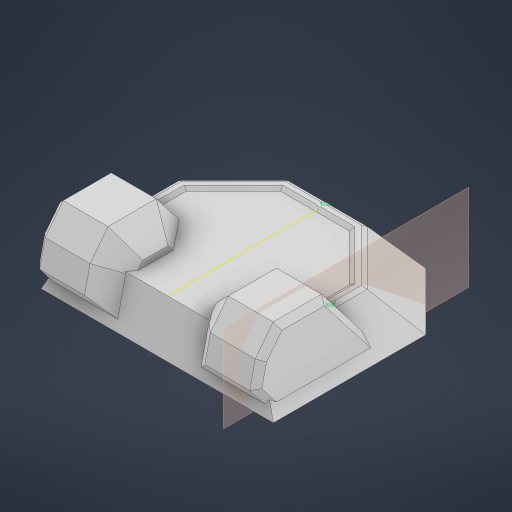
# Autodesk Inventor part: chassis
Saved by Autodesk Inventor 2023 (Build 270158000, 158)
## iProperties
Created: 2022-06-22
Part Number: chassis
Material: Generic
Document SubType Name: Modeling
Designer: Dan
Density: 1 g/cm^3
Appearance: Default
Author: Dan
Autodesk Inventor part; units mm, degrees
ref_plane "XY Plane" through (0, 0, 0) normal (0, 0, 1) x (1, 0, 0)
sketch "Sketch2" plane through (0, 0, 0) normal (0, 1, 0) x (-1, 0, 0)
  line L0 (0, -90) -> (0, 90)
  line L1 (0, -90) -> (-50, -90)
  line L2 (-50, -90) -> (-99.4975, -40.5025)
  line L3 (-99.4975, -40.5025) -> (-99.4975, 90)
  line L4 (-99.4975, 90) -> (0, 90)
  point P0 (0, 0)
  dimension "d0" = 180
  dimension "d1" = 50
  dimension "d2" = 70
  dimension "d3" = 135
  constraints: 10 end point, 2 midpoint, 2 perpendicular, 1 horizontal, 1 vertical
  measures "d0" distance of L0.start L0.end
  measures "d1" distance of L0.start L1.end
  measures "d2" distance of L1.end L2.end
  measures "d3" angle of L1 L2
ref_plane "Top" through (0, 40, 0) normal (0, 1, 0) x (-1, 0, 0)
sketch "Sketch3" plane through (0, 40, 0) normal (0, 1, 0) x (-1, 0, 0)
  line L0 (0, -90) -> (0, 90) projected
  line L1 (0, -90) -> (-50, -90) projected
  line L2 (-50, -90) -> (-99.4975, -40.5025) projected
  line L3 (-99.4975, -40.5025) -> (-99.4975, 90) projected
  line L4 (-99.4975, 90) -> (0, 90) projected
  line L5 (-34.0658, -55.9075) -> (0, -55.9075)
  line L6 (0, 81.0844) -> (-80.6502, 81.0844)
  line L7 (-80.6502, 81.0844) -> (-80.6502, -9.3231)
  line L8 (-80.6502, -9.3231) -> (-34.0658, -55.9075)
  point P0 (0, 0)
  constraints: 8 end point, 4 parallel, 2 point on line, 1 horizontal, 1 vertical
loft "Loft1" add profiles "Sketch2", "Sketch3" contours all / L5 L8 L7 L6 L0
ref_plane "WHeel" through (60, 0, -90) normal (-1, 0, 0) x (0, 0, 1)
sketch "Sketch4" plane through (60, 0, -90) normal (-1, 0, 0) x (0, 0, 1)
  line L0 (49.4975, 0) -> (180, 0) projected
  line L1 (150, -2) -> (150, 63) construction
  circle A0 centre (150, 30.5) radius 32.5
  point P0 (90, 0)
  dimension "wheeld" = 65
  dimension "rideh" = 2
  dimension "d14" = 65
  dimension "d17" = 30
  constraints: 2 end point, 1 centre point, 1 midpoint, 1 vertical
  measures "wheeld" distance of L1.start L1.end
  measures "rideh" distance from line of L1.start L0
  measures "d14" diameter of A0
  measures "d17" distance from line of L0.end L1
extrude "Extrusion1" add sketch "Sketch4" against normal blind 35 separate body
sketch "Sketch5" plane through (95, 30.5, 60) normal (1, 0, 0) x (0, 0, -1)
  circle A0 centre (0, 0) radius 32.5 projected
  line L0 (-20.6148, 34.967) -> (20.6148, 34.967)
  line L1 (20.6148, 34.967) -> (71.6455, -30.5)
  line L2 (-30, -30.5) -> (100.5025, -30.5) projected
  line L3 (100.5025, -30.5) -> (69.3231, 9.5) projected
  circle A1 centre (0, 0) radius 32.5 projected
  line L4 (0, 32.5) -> (0, 40.0339) construction
  line L5 (-20.6148, 34.967) -> (-36.015, 15.2102)
  line L6 (-40.7271, -5.9307) -> (-21.5757, -30.5)
  line L7 (-36.015, 15.2102) -> (-40.7271, -5.9307)
  line L8 (-41.2569, -30.5) -> (-31.8085, 11.8903) projected
  line L9 (71.6455, -30.5) -> (-21.5757, -30.5)
  point P0 (60, -30.5)
  point P1 (0, 34.967)
  point P2 (-21.0844, 9.5)
  dimension "d18" = 127.936
  dimension "d19" = 127.936
  constraints: 14 end point, 4 point on line, 2 parallel, 1 collinear, 1 horizontal, 1 midpoint, 1 vertical, 1 vertical alignment, 1 other
  measures "d18" angle of L0 L1
  measures "d19" angle of L5 L0
extrude "Extrusion2" add sketch "Sketch5" against normal blind 63.5 separate body contours A0 L2 | A0 L2 L6 L7 L5 L0 L1 picked at (-8.2922, 7.0851)
chamfer "Chamfer1" distance 20 angle 45 4 edges at (31.5, 32.7335, 13.8699) (31.5, 65.467, 60) (31.5, 35.1397, 98.371) (31.5, 55.5886, 88.3149)
chamfer "Chamfer2" distance 5 angle 45 5 edges at (95, 32.7335, 13.8699) (95, 65.467, 60) (95, 55.5886, 88.3149) (95, 35.1397, 98.371) (95, 12.2846, 91.1514)
ref_plane "Work Plane3" through (0, 42, 81.0844) normal (0, 1, 0) x (1, 0, 0)
sketch "Sketch7" plane through (0, 42, 81.0844) normal (0, 1, 0) x (1, 0, 0)
  line L0 (34.0658, 136.9919) -> (0, 136.9919) projected
  line L1 (80.6502, 90.4075) -> (34.0658, 136.9919) projected
  line L2 (80.6502, 0) -> (80.6502, 90.4075) projected
  line L3 (0, 0) -> (80.6502, 0) projected
  line L4 (31.9947, 131.9919) -> (77.6502, 86.3364)
  line L5 (77.6502, 86.3364) -> (77.6502, 3)
  line L6 (77.6502, 3) -> (0, 3)
  line L7 (31.9947, 131.9919) -> (0, 131.9919)
  line L8 (0, 171.0844) -> (0, -8.9156) projected
  line L9 (0, 136.9919) -> (0, 0) projected
  point P0 (0, 81.0844)
  dimension "d37" = 5
  dimension "d38" = 5
  dimension "d39" = 3
  constraints: 8 end point, 1 parallel, 1 other
  measures "d37" distance between parallel lines of L1 L4
  measures "d38" distance between parallel lines of L0 L7
  measures "d39" distance between parallel lines of L2 L5
sketch "Sketch6" plane through (31.5, 30.5, 60) normal (-1, 0, 0) x (0, 0, 1)
  line L0 (-46.2872, -30.5) -> (21.5757, -30.5) projected
  line L1 (17.4734, 6.4652) -> (24.7927, -26.3729) projected
  line L2 (-10.8463, 14.967) -> (10.8463, 14.967) projected
  line L3 (-46.2872, -30.5) -> (-10.8463, 14.967) projected
  line L4 (-46.2872, -30.5) -> (21.5757, -30.5) projected
  line L5 (21.5757, -30.5) -> (24.7927, -26.3729) projected
  line L6 (10.8463, 14.967) -> (17.4734, 6.4652) projected
  point P0 (-60, -30.5)
  point P1 (-46.2872, -30.5)
extrude "Extrusion3" [suppressed]
combine bodies "Combine1" operation type add bodies to combine 3 1
shell "Shell1" thickness 3 removed faces 1 at (0, 3.3333, 15.7504) bodies 3
sketch "Sketch8" plane through (0, 0, -90) normal (-1, 0, 0) x (0, 0, 1)
  line L0 (80.6769, 40) -> (34.0925, 40) projected
  line L1 (34.0925, 40) -> (37.5566, 42)
  line L2 (41.5566, 42) -> (37.5566, 42)
  line L3 (34.0925, 40) -> (171.0844, 40) projected
  line L4 (0, 0) -> (34.0925, 40) projected
  line L5 (39.5566, 42) -> (39.5566, 40)
  line L6 (45.0207, 40) -> (41.5566, 42)
  point P0 (90, 0)
  dimension "d46" = 30
  dimension "d47" = 2
  dimension "d48" = 4
  constraints: 8 end point, 1 horizontal, 1 midpoint, 1 point on line, 1 symmetric about line, 1 vertical
  measures "d46" angle of L0 L1
  measures "d47" distance between parallel lines of L0 L2
  measures "d48" distance of L2.start L1.end
sketch3d "3D Sketch1"
  line L0 (0, 40, -55.9075) -> (34.0658, 40, -55.9075)
  line L1 (34.0658, 40, -55.9075) -> (80.6502, 40, -9.3231)
  line L2 (80.6502, 40, -9.3231) -> (80.6502, 40, 19.534)
sweep "Sweep1" add profiles "Sketch8" path "3D Sketch1" bodies 3
ref_plane "Work Plane4" through (77.1861, 42, 19.534) normal (1, 0, 0) x (0, 1, 0)
sketch "Sketch9" plane through (77.1861, 42, 19.534) normal (1, 0, 0) x (0, 1, 0)
  line L0 (-2, 0) -> (-2, -28.8571) projected
  line L1 (-2, -3.9347) -> (0, -0.4706)
  line L2 (0, -0.4706) -> (0, 2.2891)
  line L3 (0, 2.2891) -> (-2, 2.2891)
  line L4 (-2, 2.2891) -> (-2, -3.9347)
  point P0 (-42, -19.534)
  dimension "d51" = 30
  dimension "d52" = 2
  constraints: 8 end point, 1 collinear, 1 perpendicular, 1 point on line, 1 vertical
  measures "d51" angle of L0 L1
  measures "d52" distance from line of L0 L1.end
thicken "Thicken1" operation add thickness 2 both sides no extend neighbours no toward (0, 0, 1) bodies 3 faces at (74.5194, 40.6667, 19.534)
mirror "Mirror1" about plane through (0, 0, 0) normal (1, 0, 0) bodies 3
equation "\"d14\" = wheeld"
equation "\"d19\" = d18"
body "Solid3"
